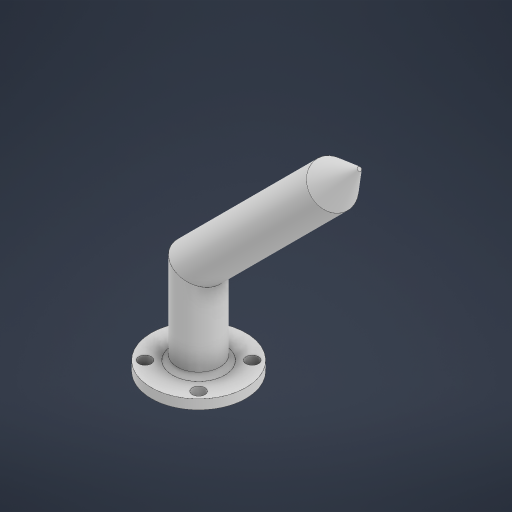
# Autodesk Inventor part: Herramienta1-2
Saved by Autodesk Inventor 2023.4 (Build 274418000, 418)
## iProperties
Created: 2024-02-24
Part Number: Herramienta1-2
Material: Generic
Document SubType Name: Modeling
Designer: ASUS
Density: 1 g/cm^3
Appearance: Default
Author: ASUS
Autodesk Inventor part; units mm, degrees
ref_plane "YZ Plane" through (0, 0, 0) normal (1, 0, 0) x (0, 1, 0)
ref_plane "XZ Plane" through (0, 0, 0) normal (0, 1, 0) x (-1, 0, 0)
ref_plane "XY Plane" through (0, 0, 0) normal (0, 0, 1) x (1, 0, 0)
sketch "Sketch1" plane through (0, 0, 0) normal (0, 0, 1) x (1, 0, 0)
  line L0 (0, 0) -> (0, 50)
  line L1 (0, 50) -> (70.7107, 120.7107)
  line L2 (0, 50) -> (30.994, 50) construction
  line L3 (70.7107, 120.7107) -> (84.8528, 134.8528) construction
  dimension "d0" = 50
  dimension "d1" = 100
  dimension "d2" = 45
  dimension "d24" = 120
  constraints: 8 end point, 1 coincident, 1 collinear, 1 horizontal, 1 vertical
  measures "d0" distance of L0.start L0.end
  measures "d1" distance of L0.end L1.end
  measures "d2" angle of L2 L1
  measures "d24" distance of L3.end L0.end
sketch "Sketch2" plane through (0, 0, 0) normal (0, 1, 0) x (-1, 0, 0)
  circle A0 centre (0, 0) radius 11.25
  circle A1 centre (0, 0) radius 8.75 construction
  dimension "d6" = 17.5
  dimension "d7" = 2.5
  dimension "d27" = 22.5
  constraints: 2 centre point, 2 coincident
  measures "d6" diameter of A1
  measures "d7" radial gap between concentric circles of A0 A1
  measures "d27" diameter of A0
sweep "Sweep1" add profiles "Sketch2" path "Sketch1"
sketch "Sketch3" plane through (0, 0, 0) normal (0, 1, 0) x (-1, 0, 0)
  circle A0 centre (0, 0) radius 11.25 projected
  circle A1 centre (0, 0) radius 20 construction
  circle A2 centre (0, 0) radius 25
  dimension "d8" = 40
  dimension "d9" = 5
  dimension "d10" = 50
  constraints: 2 centre point, 2 coincident
  measures "d8" diameter of A1
  measures "d9" radial gap between concentric circles of A2 A1
  measures "d10" diameter of A2
extrude "Extrusion1" add sketch "Sketch3" along normal blind 5
sketch "Sketch4" plane through (0, 5, 0) normal (0, 1, 0) x (1, 0, 0)
  circle A0 centre (0, 0) radius 20 construction
  point P0 (-14.1421, 14.1421)
  point P1 (-14.1421, -14.1421)
  point P2 (14.1421, -14.1421)
  point P3 (14.1421, 14.1421)
  constraints: 4 point on circle
hole "Hole1" at (-14.1421, 5, -14.1421) at (14.1421, 5, -14.1421) at (-14.1421, 5, 14.1421) at (14.1421, 5, 14.1421) direction (0, -1, 0) diameter 6.6 end through all
fillet "Fillet1" radius 2.5 1 edges at (11.25, 5, 0)
ref_plane "Work Plane1" through (84.8528, 134.8528, 0) normal (0.7071068, 0.7071068, 0) x (-0.7071068, 0.7071068, 0)
sketch "Sketch8" plane through (84.8528, 134.8528, 0) normal (0.7071068, 0.7071068, 0) x (-0.7071068, 0.7071068, 0)
  circle A0 centre (0, 0) radius 1
  point P0 (-35.3553, 0)
  dimension "d34" = 2
  constraints: 1 centre point, 1 coincident
  measures "d34" diameter of A0
loft "Loft2" add profiles "Sketch8" section 1 edges at (78.6656, 112.7557, 0)
body "Solid1"
